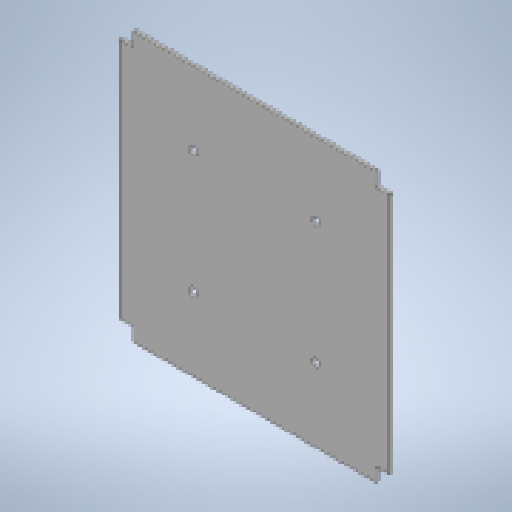
# Autodesk Inventor part: PCB_COM_BAT
Saved by Autodesk Inventor 2024 (Build 280153000, 153)
## iProperties
Created: 2023-06-28
Part Number: PCB_COM_BAT
Material: Genérico
Document SubType Name: Modeling
Designer: Personal
Density: 1 g/cm^3
Appearance: Valor por defecto
Author: Personal
Autodesk Inventor part; units mm, degrees
ref_plane "YZ Plane" through (0, 0, 0) normal (1, 0, 0) x (0, 1, 0)
ref_plane "XZ Plane" through (0, 0, 0) normal (0, 1, 0) x (-1, 0, 0)
ref_plane "XY Plane" through (0, 0, 0) normal (0, 0, 1) x (1, 0, 0)
sketch "Boceto1" plane through (0, 0, 0) normal (0, 0, 1) x (1, 0, 0)
  line L0 (-121.9033, -49.2033) -> (40.2033, -49.2033) projected
  line L1 (40.2033, -49.2033) -> (40.2033, -40.2033) projected
  line L2 (40.2033, -40.2033) -> (49.2033, -40.2033) projected
  line L3 (49.2033, -40.2033) -> (49.2033, 121.9033) projected
  line L4 (49.2033, 121.9033) -> (40.2033, 121.9033) projected
  line L5 (40.2033, 121.9033) -> (40.2033, 130.9033) projected
  line L6 (40.2033, 130.9033) -> (-121.9033, 130.9033) projected
  line L7 (-121.9033, 130.9033) -> (-121.9033, 121.9033) projected
  line L8 (-130.9033, 121.9033) -> (-130.9033, -40.2033) projected
  line L9 (-121.9033, 121.9033) -> (-130.9033, 121.9033) projected
  line L10 (-130.9033, -40.2033) -> (-121.9033, -40.2033) projected
  line L11 (-121.9033, -40.2033) -> (-121.9033, -49.2033) projected
  circle A0 centre (0, 0) radius 2.5 projected
  circle A1 centre (-81.7, 0) radius 2.8882 projected
  circle A2 centre (0, 81.7) radius 2.5 projected
  circle A3 centre (-81.7, 81.7) radius 2.8882 projected
  point P0 (0, 0)
extrude "Extrusión2" add sketch "Boceto1" along normal blind 1.65
